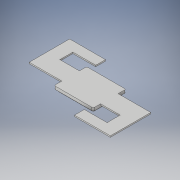
# Autodesk Inventor part: Enclosure_Top V6
Saved by Autodesk Inventor 2017 (Build 210142000, 142)
## iProperties
Created: 2017-12-18
Part Number: Enclosure_Top V6
Material: Generic
Document SubType Name: Modeling
Designer: Tripl_000
Density: 1 g/cm^3
Appearance: Default
Author: Tripl_000
Autodesk Inventor part; units mm, degrees
ref_plane "YZ Plane" through (0, 0, 0) normal (1, 0, 0) x (0, 1, 0)
ref_plane "XZ Plane" through (0, 0, 0) normal (0, 1, 0) x (-1, 0, 0)
ref_plane "XY Plane" through (0, 0, 0) normal (0, 0, 1) x (1, 0, 0)
sketch "Sketch1" plane through (0, 0, 0) normal (0, 1, 0) x (-1, 0, 0)
  line L0 (27.75, 22.75) -> (-27.75, 22.75)
  line L1 (-27.75, 22.75) -> (-27.75, -22.75)
  line L2 (-27.75, -22.75) -> (27.75, -22.75)
  line L3 (27.75, -22.75) -> (27.75, 22.75)
  line L4 (27.75, 22.75) -> (-27.75, -22.75) construction
  line L5 (-27.75, 22.75) -> (27.75, -22.75) construction
  point P0 (0, 0)
  dimension "d0" = 55.5
  dimension "d1" = 45.5
  constraints: 12 end point, 2 midpoint, 2 parallel, 1 horizontal, 1 perpendicular
  measures "d0" distance of L0.start L0.end
  measures "d1" distance of L2.end L0.start
extrude "Extrusion1" add sketch "Sketch1" along normal blind 2.5
sketch "Sketch2" plane through (0, 2.5, 0) normal (0, 1, 0) x (1, 0, 0)
  line L0 (-30, -25) -> (30, -25)
  line L1 (30, -25) -> (30, 25)
  line L2 (30, 25) -> (-30, 25)
  line L3 (-30, 25) -> (-30, -25)
  line L4 (-30, -25) -> (30, 25) construction
  line L5 (30, -25) -> (-30, 25) construction
  point P0 (0, 0)
  dimension "d4" = 50
  dimension "d5" = 60
  constraints: 12 end point, 2 midpoint, 2 parallel, 1 horizontal, 1 perpendicular
  measures "d4" distance of L2.end L0.start
  measures "d5" distance of L0.start L0.end
extrude "Extrusion2" add sketch "Sketch2" along normal blind 2.5
sketch "Sketch3" plane through (27.75, 0, 22.75) normal (1, 0, 0) x (0, 0, -1)
  line L0 (16.25, -2.5) -> (29.25, -2.5)
  line L1 (29.25, -2.5) -> (29.25, 2.5)
  line L2 (29.25, 2.5) -> (16.25, 2.5)
  line L3 (16.25, 2.5) -> (16.25, -2.5)
  line L4 (16.25, -2.5) -> (29.25, 2.5) construction
  line L5 (29.25, -2.5) -> (16.25, 2.5) construction
  point P0 (22.75, 0)
  dimension "d8" = 13
  dimension "d9" = 5
  constraints: 12 end point, 2 midpoint, 2 parallel, 1 horizontal, 1 perpendicular
  measures "d8" distance of L1.end L2.end
  measures "d9" distance of L0.end L1.end
extrude "Extrusion3" cut sketch "Sketch3" against normal through all
sketch "Sketch4" plane through (0, 5, 0) normal (0, 1, 0) x (1, 0, 0)
  line L0 (0, 31.16) -> (0, -35.6529)
  line L1 (-50.8705, 0) -> (45.6531, 0)
  circle A0 centre (-25, 20) radius 1.5
  circle A1 centre (25, 20) radius 1.5
  circle A2 centre (-25, -20) radius 1.5
  circle A3 centre (25, -20) radius 1.5
  point P0 (0, 0)
  dimension "d12" = 25
  dimension "d13" = 20
  dimension "d14" = 3
  constraints: 4 centre point, 4 end point, 3 symmetric about line, 1 horizontal, 1 vertical, 3 other
  measures "d12" horizontal distance of point (0, 0) A0.centre
  measures "d13" vertical distance of point (0, 0) A0.centre
  measures "d14" diameter of A0
extrude "Extrusion4" cut sketch "Sketch4" against normal through all
fillet "Fillet1" radius 2 8 edges at (-27.75, 1.25, 22.75) (27.75, 1.25, 22.75) (27.75, 1.25, -22.75) (-27.75, 1.25, -22.75) (-30, 3.75, -25) (-30, 3.75, 25) (30, 3.75, 25) (30, 3.75, -25)
sketch "Sketch5" plane through (30, 2.5, 23) normal (1, 0, 0) x (0, 0, -1)
  line L0 (46, 0) -> (0, 0) projected
  line L1 (0, 2.5) -> (46, 2.5) projected
  line L2 (16.75, 0) -> (29.25, 0)
  line L3 (29.25, 0) -> (29.25, 2.5)
  line L4 (29.25, 2.5) -> (16.75, 2.5)
  line L5 (16.75, 2.5) -> (16.75, 0)
  line L6 (29.5, 0) -> (29.5, -2.5) projected
  point P0 (23, -2.5)
  dimension "d18" = 12.5
  dimension "d90" = 0.25
  constraints: 8 end point, 2 parallel, 2 point on line, 1 horizontal, 1 perpendicular
  measures "d18" distance between parallel lines of L5 L3
  measures "d90" distance between parallel lines of L6 L3
extrude "Extrusion5" add sketch "Sketch5" along normal blind 32
ref_plane "Work Plane1" through (0, 2.5, -23) normal (1, 0, 0) x (0, 0, -1)
mirror "Mirror1" about plane through (0, 2.5, -23) normal (1, 0, 0) of "Extrusion5"
sketch "Sketch6" plane through (-62, 2.5, 6.25) normal (-1, 0, 0) x (0, 0, 1)
  line L0 (0, 0) -> (-12.5, 0) projected
  line L1 (-9, 2.5) -> (-3.5, 2.5)
  line L2 (-3.5, 2.5) -> (-3.5, 0)
  line L3 (-3.5, 0) -> (-9, 0)
  line L4 (-9, 0) -> (-9, 2.5)
  line L5 (-12.5, 0) -> (-12.5, 2.5) projected
  line L6 (0, 2.5) -> (0, 0) projected
  line L7 (-12.5, 2.5) -> (0, 2.5) projected
  point P0 (-6.25, -2.5)
  dimension "d23" = 3.5
  dimension "d24" = 3.5
  dimension "d25" = 0
  constraints: 8 end point, 2 parallel, 1 horizontal, 1 perpendicular, 1 point on line
  measures "d23" distance between parallel lines of L5 L4
  measures "d24" distance between parallel lines of L6 L2
  measures "d25" distance between parallel lines of L7 L1
extrude "Extrusion6" add sketch "Sketch6" along normal blind 17.5 contours L0 L4 L1 L2
mirror "Mirror2" about plane through (0, 2.5, -23) normal (1, 0, 0) of "Extrusion6"
sketch "Sketch7" plane through (62, 2.5, 2.75) normal (0, 0, 1) x (1, 0, 0)
  line L0 (0, 2.5) -> (17.5, 2.5) projected
  line L1 (0, 0) -> (17.5, 0) projected
  line L2 (15.5, 2.5) -> (9, 2.5)
  line L3 (9, 2.5) -> (9, 0)
  line L4 (9, 0) -> (15.5, 0)
  line L5 (15.5, 2.5) -> (15.5, 0)
  line L6 (0, 0) -> (17.5, 0) projected
  point P0 (-62, -2.5)
  constraints: 8 end point, 2 perpendicular, 2 point on line, 1 horizontal, 1 parallel
extrude "Extrusion7" add sketch "Sketch7" along normal blind 43
sketch "Sketch8" plane through (71, 2.5, 2.75) normal (-1, 0, 0) x (0, 0, 1)
  line L0 (43, 2.5) -> (43, 0) projected
  line L1 (0, 0) -> (43, 0) projected
  line L2 (43, 2.5) -> (34, 2.5)
  line L3 (34, 2.5) -> (34, 0)
  line L4 (34, 0) -> (43, 0)
  line L5 (43, 0) -> (43, 2.5)
  point P0 (-2.75, -2.5)
  dimension "d31" = 9
  constraints: 8 end point, 2 parallel, 1 horizontal, 1 perpendicular, 1 point on line
  measures "d31" distance between parallel lines of L0 L3
extrude "Extrusion8" add sketch "Sketch8" along normal blind 43.5
sketch "Sketch9" plane through (-62, 2.5, -2.75) normal (0, 0, -1) x (-1, 0, 0)
  line L0 (0, 2.5) -> (17.5, 2.5) projected
  line L1 (0, 0) -> (17.5, 0) projected
  line L2 (15.5, 2.5) -> (9, 2.5)
  line L3 (9, 2.5) -> (9, 0)
  line L4 (9, 0) -> (15.5, 0)
  line L5 (0, 2.5) -> (17.5, 2.5) projected
  line L6 (15.5, 2.5) -> (15.5, 0)
  line L7 (17.5, 2.5) -> (17.5, 0) projected
  point P0 (-62, -2.5)
  dimension "d96" = 2
  constraints: 8 end point, 2 perpendicular, 2 point on line, 1 horizontal, 1 parallel
  measures "d96" distance between parallel lines of L7 L6
extrude "Extrusion9" add sketch "Sketch9" along normal blind 43 contours L0 L6 L1 L3
sketch "Sketch10" plane through (-71, 2.5, -2.75) normal (1, 0, 0) x (0, 0, -1)
  line L0 (43, 2.5) -> (43, 0) projected
  line L1 (0, 2.5) -> (43, 2.5) projected
  line L2 (43, 0) -> (34, 0)
  line L3 (34, 0) -> (34, 2.5)
  line L4 (34, 2.5) -> (43, 2.5)
  line L5 (43, 2.5) -> (43, 0)
  point P0 (-2.75, -2.5)
  dimension "d37" = 9
  constraints: 8 end point, 2 parallel, 1 horizontal, 1 perpendicular, 1 point on line
  measures "d37" distance between parallel lines of L0 L3
extrude "Extrusion10" add sketch "Sketch10" along normal blind 43.5
fillet "Fillet2" radius 7.5 4 edges at (-71, 3.75, -2.75) (-71, 3.75, -36.75) (71, 3.75, 36.75) (71, 3.75, 2.75)
fillet "Fillet3" radius 5 4 edges at (62, 3.75, 6.25) (62, 3.75, -6.25) (-62, 3.75, -6.25) (-62, 3.75, 6.25)
sketch "Sketch11" plane through (0, 5, 0) normal (0, 1, 0) x (1, 0, 0)
  line L0 (28, -25) -> (-28, -25)
  line L1 (-28, 25) -> (28, 25)
  line L2 (30, -25) -> (-30, 25) construction
  line L3 (-30, -25) -> (30, 25) construction
  arc A0 (28, -25) -> (30, -23) centre (28, -23) ccw
  arc A1 (-30, -23) -> (-28, -25) centre (-28, -23) ccw
  arc A2 (-28, 25) -> (-30, 23) centre (-28, 23) ccw
  arc A3 (30, 23) -> (28, 25) centre (28, 23) ccw
  line L4 (-30, -13.25) -> (-80, -13.25)
  line L5 (-80, -13.25) -> (-80, 48.75)
  line L6 (-80, 48.75) -> (-25, 48.75)
  line L7 (-25, 48.75) -> (-25, 33.75)
  line L8 (-25, 33.75) -> (-60, 33.75)
  line L9 (-60, 33.75) -> (-60, 13.75)
  line L10 (-60, 13.75) -> (-30, 13.75)
  line L11 (-30, 23) -> (-30, 6.25) projected
  line L12 (30, -13.75) -> (60, -13.75)
  line L13 (60, -13.75) -> (60, -33.75)
  line L14 (60, -33.75) -> (25, -33.75)
  line L15 (25, -33.75) -> (25, -48.75)
  line L16 (25, -48.75) -> (80, -48.75)
  line L17 (80, -48.75) -> (80, 13.25)
  line L18 (80, 13.25) -> (30, 13.25)
  line L19 (-30, -6.25) -> (-62, -6.25) projected
  line L20 (30, 6.25) -> (62, 6.25) projected
  line L21 (30, 23) -> (30, 13.25)
  line L22 (30, -13.75) -> (30, -23)
  line L23 (-30, -23) -> (-30, -13.25)
  line L24 (-30, 13.75) -> (-30, 23)
  point P0 (0, 0)
  point P1 (-57.2303, -6.25)
  point P2 (57.2303, 6.25)
  dimension "d42" = 2
  dimension "d43" = 50
  dimension "d44" = 50
  dimension "d45" = 27
  dimension "d46" = 7
  dimension "d47" = 7
  dimension "d48" = 27
  dimension "d49" = 20
  dimension "d50" = 20
  dimension "d51" = 15
  dimension "d52" = 15
  dimension "d53" = 20
  dimension "d54" = 20
  dimension "d55" = 55
  dimension "d56" = 55
  constraints: 46 end point, 16 perpendicular, 12 tangent, 8 point on circle, 5 parallel, 5 point on line, 4 centre point, 3 equal radius, 3 horizontal, 2 midpoint
  measures "d42" radius of A0
  measures "d43" distance of L4.start L4.end
  measures "d44" distance of L18.end L17.end
  measures "d45" distance between parallel lines of L10 L4
  measures "d46" distance between parallel lines of L19 L4
  measures "d47" distance between parallel lines of L18 L20
  measures "d48" distance between parallel lines of L18 L12
  measures "d49" distance between parallel lines of L5 L9
  measures "d50" distance between parallel lines of L13 L17
  measures "d51" distance between parallel lines of L14 L16
  measures "d52" distance between parallel lines of L6 L8
  measures "d53" distance of L8.end L9.end
  measures "d54" distance of L12.end L13.end
  measures "d55" distance of L15.end L16.end
  measures "d56" distance of L5.end L6.end
extrude "Extrusion11" add sketch "Sketch11" along normal blind 2
ref_plane "Work Plane2" through (0, 0, 0) normal (0, -1, 0) x (1, 0, 0)
sketch "Sketch15" plane through (0, 0, 0) normal (0, -1, 0) x (1, 0, 0)
  line L0 (-86.692, 0) -> (98.0849, 0)
  circle A0 centre (-25, -20) radius 1.5 projected
  circle A1 centre (-25, -20) radius 2
  circle A2 centre (25, -20) radius 1.5 projected
  circle A3 centre (25, -20) radius 2
  circle A4 centre (-25, 20) radius 2
  circle A5 centre (25, 20) radius 2
  point P0 (0, 0)
  dimension "d91" = 4
  dimension "d92" = 4
  constraints: 4 centre point, 2 coincident, 2 end point, 2 symmetric about line, 1 horizontal, 2 other
  measures "d91" diameter of A1
  measures "d92" diameter of A3
extrude "Extrusion15" add sketch "Sketch15" against normal up to surface (7 mm away) contours A0 | A1 | A2 | A3 | A4 | A5
sketch "Sketch16" plane through (79.5, 2.5, -2.75) normal (0, 0, -1) x (-1, 0, 0)
  line L0 (2, 0) -> (0, 0) projected
  line L1 (17.5, 2.5) -> (0, 2.5) projected
  line L2 (0, 0) -> (2, 0)
  line L3 (2, 0) -> (2, 2.5)
  line L4 (2, 2.5) -> (0, 2.5)
  line L5 (0, 2.5) -> (0, 0)
  point P0 (79.5, -2.5)
  dimension "d98" = 2
  constraints: 8 end point, 2 parallel, 1 horizontal, 1 perpendicular, 1 point on line
  measures "d98" distance between parallel lines of L5 L3
extrude "Extrusion16" cut sketch "Sketch16" against normal through all
sketch "Sketch17" plane through (-77.5, 2.5, -2.75) normal (0, 0, -1) x (-1, 0, 0)
  line L0 (-15.5, 0) -> (2, 0) projected
  line L1 (2, 0) -> (0, 0)
  line L2 (0, 0) -> (0, 2.5)
  line L3 (0, 2.5) -> (2, 2.5)
  line L4 (2, 2.5) -> (2, 0)
  point P0 (-77.5, -2.5)
  constraints: 8 end point, 2 parallel, 1 horizontal, 1 perpendicular
extrude "Extrusion17" cut sketch "Sketch17" against normal through all
fillet "Fillet4" radius 7.5 4 edges at (77.5, 3.75, -2.75) (77.5, 3.75, 45.75) (-77.5, 3.75, 2.75) (-77.5, 3.75, -45.75)
body "Solid1"
